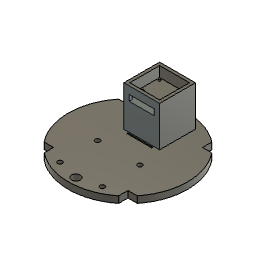
cam_mount v6 (Autodesk Fusion 360 design; units mm, degrees)
Autodesk Fusion 360 part; units mm, degrees
sketch "Sketch1" plane through (0, 0, 0) normal (0, 1, 0) x (1, 0, 0)
  arc A0 (31.75, 39.6557) -> (-31.75, 39.6557) centre (0, 0) ccw
  arc A1 (39.6557, -31.75) -> (39.6557, 31.75) centre (0, 0) ccw
  arc A2 (-39.6557, 31.75) -> (-39.6557, -31.75) centre (0, 0) ccw
  arc A3 (-31.75, -39.6557) -> (31.75, -39.6557) centre (0, 0) ccw
  line L0 (-31.75, -39.6557) -> (-31.75, -31.75)
  line L1 (-31.75, 31.75) -> (-31.75, 39.6557)
  line L2 (39.6557, 31.75) -> (31.75, 31.75)
  line L3 (-31.75, 31.75) -> (-39.6557, 31.75)
  line L4 (31.75, 39.6557) -> (31.75, 31.75)
  line L5 (31.75, -31.75) -> (31.75, -39.6557)
  line L6 (-39.6557, -31.75) -> (-31.75, -31.75)
  line L7 (31.75, -31.75) -> (39.6557, -31.75)
  dimension "d1" = 101.6
  constraint coincident A0.centre A1.centre
  constraint vertical L4
  constraint vertical L0
  constraint horizontal L2
  constraint horizontal L6
  constraint concentric A0 A2
  constraint concentric A1 A2
  constraint concentric A2 A3
  constraint coincident L1.start L2
  constraint collinear L0 L1
  constraint collinear L2 L3
  constraint coincident L5.start L6
  constraint collinear L4 L5
  constraint collinear L6 L7
  measures "d1" diameter of A2
sketch "Sketch2" plane through (0, 0, 0) normal (0, 1, 0) x (1, 0, 0)
  circle A0 centre (-18.034, -7.874) radius 2.032
  circle A1 centre (18.034, -7.874) radius 2.032
  circle A2 centre (-18.034, -39.878) radius 2.032
  circle A3 centre (18.034, -39.878) radius 2.032
  dimension "d9" = 36.068
  dimension "d11" = 32.004
  dimension "d12" = 36.068
  dimension "d13" = 4.064
  dimension "d14" = 4.064
  dimension "d15" = 4.064
  dimension "d16" = 4.064
  measures "d9" distance of A2.centre A3.centre
  measures "d11" distance of A0.centre A2.centre
  measures "d12" distance of A0.centre A1.centre
  measures "d13" diameter of A0
  measures "d14" diameter of A1
  measures "d15" diameter of A2
  measures "d16" diameter of A3
extrude "Extrude1" add sketch "Sketch1" against normal blind 5.588
sketch "Sketch4" plane through (0, 0, 0) normal (0, 1, 0) x (1, 0, 0)
  circle A0 centre (18.034, -39.878) radius 2.032
  line L0 (12.7, 39.6369) -> (12.7, 14.2369)
  line L1 (15.24, 11.6969) -> (-15.24, 11.6969)
  line L2 (-12.7, 14.2369) -> (-12.7, 39.6369)
  line L3 (15.24, 42.1769) -> (15.24, 11.6969)
  line L4 (12.7, 14.2369) -> (-12.7, 14.2369)
  circle A1 centre (18.034, -7.874) radius 2.032
  line L5 (-15.24, 42.1769) -> (15.24, 42.1769)
  circle A2 centre (-18.034, -39.878) radius 2.032
  line L6 (-12.7, 39.6369) -> (12.7, 39.6369)
  circle A3 centre (-18.034, -7.874) radius 2.032
  line L7 (-15.24, 11.6969) -> (-15.24, 42.1769)
  dimension "d29" = 36.068
  dimension "d30" = 32.004
  dimension "d31" = 36.068
  dimension "d32" = 4.064
  dimension "d33" = 4.064
  dimension "d34" = 4.064
  dimension "d35" = 4.064
  constraint horizontal L5
  constraint vertical L3
  constraint horizontal L1
  constraint vertical L7
  constraint horizontal L4
  constraint vertical L2
  constraint horizontal L6
  constraint vertical L0
  measures "d29" distance of A0.centre A2.centre
  measures "d30" distance of A3.centre A2.centre
  measures "d31" distance of A3.centre A1.centre
  measures "d32" diameter of A3
  measures "d33" diameter of A1
  measures "d34" diameter of A2
  measures "d35" diameter of A0
extrude "Extrude2" cut sketch "Sketch2" against normal blind 22
extrude "Extrude3" add sketch "Sketch4" along normal blind 34.29 contours L1 L3 L5 L7
extrude "Extrude4" add 1 faces at (-4.2333, 0, -31.1702) along direction (0, 1, 0) blind 25.4
sketch "Sketch5" plane through (0, 25.4, 0) normal (0, 1, 0) x (-1, 0, 0)
  line L0 (12.7, -14.2369) -> (-12.7, -14.2369)
  line L1 (-12.7, -14.2369) -> (-12.7, -39.6369)
  line L2 (-12.7, -39.6369) -> (12.7, -39.6369)
  line L3 (12.7, -39.6369) -> (12.7, -14.2369)
  line L4 (12.7, -14.2369) -> (-12.7, -14.2369)
  line L5 (-12.7, -14.2369) -> (-12.7, -19.8249)
  line L6 (-12.7, -19.8249) -> (12.7, -19.8249)
  line L7 (12.7, -19.8249) -> (12.7, -14.2369)
  dimension "d42" = 5.588
  constraint horizontal L4
  constraint vertical L5
  constraint horizontal L6
  constraint vertical L7
  constraint coincident L0.start L3.end
  measures "d42" distance of L0.start L6.end
extrude "Extrude5" cut sketch "Sketch5" against normal blind 2.54 contours L0 L1 L3 L4 L5 L6 L7
sketch "Sketch6" plane through (0, 0, -14.2369) normal (0, 0, -1) x (-1, 0, 0)
  line L0 (12.7, 22.86) -> (12.7, 34.29)
  line L1 (12.7, 34.29) -> (-12.7, 34.29)
  line L2 (-12.7, 34.29) -> (-12.7, 22.86)
  line L3 (-12.7, 22.86) -> (12.7, 22.86)
  line L4 (-10.668, 27.94) -> (10.668, 27.94)
  line L5 (10.668, 27.94) -> (10.668, 22.86)
  line L6 (10.668, 22.86) -> (-10.668, 22.86)
  line L7 (-10.668, 22.86) -> (-10.668, 27.94)
  constraint horizontal L4
  constraint vertical L5
  constraint horizontal L6
  constraint vertical L7
  constraint coincident L3 L5.end
extrude "Extrude6" cut sketch "Sketch6" against normal blind 17 contours L3 L4 L5 L6 L7
sketch "Sketch7" plane through (0, 0, -11.6969) normal (0, 0, 1) x (1, 0, 0)
  line L0 (-10.668, 22.86) -> (-10.668, 27.94)
  line L1 (-10.668, 27.94) -> (10.668, 27.94)
  line L2 (10.668, 27.94) -> (10.668, 22.86)
  line L3 (10.668, 22.86) -> (-10.668, 22.86)
  line L4 (-15.24, 0) -> (15.24, 0)
  line L5 (15.24, 0) -> (15.24, 34.29)
  line L6 (15.24, 34.29) -> (-15.24, 34.29)
  line L7 (-15.24, 34.29) -> (-15.24, 0)
sketch "Sketch8" plane through (0, 25.4, 0) normal (0, 1, 0) x (-1, 0, 0)
  line L0 (12.7, -19.8249) -> (-12.7, -19.8249)
  line L1 (-12.7, -19.8249) -> (-12.7, -39.6369)
  line L2 (-12.7, -39.6369) -> (12.7, -39.6369)
  line L3 (12.7, -39.6369) -> (12.7, -19.8249)
  circle A0 centre (10.7, -37.6369) radius 1
  circle A1 centre (-10.7, -37.6369) radius 1
  circle A2 centre (10.7, -23.1369) radius 1
  circle A3 centre (-10.7, -23.1369) radius 1
  dimension "d53" = 2
  dimension "d54" = 2
  dimension "d56" = 2
  dimension "d57" = 2
  measures "d53" diameter of A0
  measures "d54" diameter of A1
  measures "d56" diameter of A2
  measures "d57" diameter of A3
extrude "Extrude7" cut sketch "Sketch8" against normal blind 4 contours A0 | A1 | A2 | A3
sketch "Sketch9" plane through (0, 0, 0) normal (0, 1, 0) x (-1, 0, 0)
  arc A0 (31.75, 39.6557) -> (-31.75, 39.6557) centre (0, 0) ccw
  line L0 (-31.75, 39.6557) -> (-31.75, 31.75)
  line L1 (-31.75, 31.75) -> (-39.6557, 31.75)
  arc A1 (-39.6557, 31.75) -> (-39.6557, -31.75) centre (0, 0) ccw
  line L2 (-39.6557, -31.75) -> (-31.75, -31.75)
  line L3 (-31.75, -31.75) -> (-31.75, -39.6557)
  arc A2 (-31.75, -39.6557) -> (31.75, -39.6557) centre (0, 0) ccw
  line L4 (31.75, -39.6557) -> (31.75, -31.75)
  line L5 (31.75, -31.75) -> (39.6557, -31.75)
  arc A3 (39.6557, -31.75) -> (39.6557, 31.75) centre (0, 0) ccw
  line L6 (39.6557, 31.75) -> (31.75, 31.75)
  line L7 (31.75, 31.75) -> (31.75, 39.6557)
  circle A4 centre (18.034, 7.874) radius 2.032
  circle A5 centre (18.034, 39.878) radius 2.032
  circle A6 centre (-18.034, 7.874) radius 2.032
  circle A7 centre (-18.034, 39.878) radius 2.032
  line L8 (15.24, -11.6969) -> (15.24, -42.1769)
  line L9 (15.24, -42.1769) -> (-15.24, -42.1769)
  line L10 (-15.24, -42.1769) -> (-15.24, -11.6969)
  line L11 (-15.24, -11.6969) -> (15.24, -11.6969)
  circle A8 centre (0, 44.3767) radius 3.6975
extrude "Extrude8" cut sketch "Sketch9" against normal blind 17 contours A8
sketch "Sketch10" plane through (0, 0, 0) normal (0, 1, 0) x (1, 0, 0)
  line L0 (-15.24, 11.6969) -> (15.24, 11.6969)
  line L1 (15.24, 10.2652) -> (14.8192, 10.2652)
  line L2 (10.668, 14.2369) -> (10.668, 11.6969)
  line L3 (-10.668, 9.8177) -> (10.2472, 9.8177)
  line L4 (10.2472, 9.8177) -> (10.2472, 10.7473)
  line L5 (10.2472, 10.7473) -> (-10.668, 10.7473)
  line L6 (-10.668, 10.7473) -> (-10.668, 9.8177)
  point P0 (-15.24, 11.6969)
  constraint horizontal L3
  constraint vertical L4
  constraint horizontal L5
  constraint vertical L6
extrude "Extrude9" cut sketch "Sketch10" against normal blind 14
